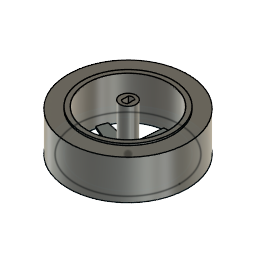
chassis_v1 (Autodesk Fusion 360 archive; units mm, degrees)
design "BO_Wheel"
part number: 2025-11-15-17-17-48-171
Autodesk Fusion 360 part; units mm, degrees
note: some values were not read from the file. Set by a fixed rule: which face or edge a step refers to.
sketch "Sketch1" plane through (0, 0, 0) normal (0, 0, 1) x (1, 0, 0)
  circle A0 centre (0, 0) radius 23.675
  circle A1 centre (0, 0) radius 23.175
  dimension "d1" = 47.35
  dimension "d2" = 46.35
  constraint coincident A0.centre A1.centre
  measures "d1" diameter of A0
  measures "d2" diameter of A1
extrude "Extrude1" add sketch "Sketch1" along normal blind 24.4 makes body 1
sketch "Sketch2" plane through (0, 0, 24.4) normal (0, 0, 1) x (-1, 0, 0)
  circle A0 centre (0, 0) radius 23.175
  circle A1 centre (0, 0) radius 23.675
  circle A2 centre (0, 0) radius 25.7
  dimension "d5" = 51.4
  constraint concentric A0 A2
  measures "d5" diameter of A2
extrude "Extrude2" add sketch "Sketch2" against normal blind 1 contours A1 | A2 bodies 1
mirror "Mirror1" about plane through (0, 0, 12.2) normal (0, 0, -1) of bodies 1 merged
sketch "Sketch3" plane through (0, 0, 1) normal (0, 0, 1) x (-1, 0, 0)
  circle A0 centre (0, 0) radius 25.7
  circle A1 centre (0, 0) radius 23.675
  circle A2 centre (0, 0) radius 33.8
  dimension "d10" = 67.6
  constraint coincident A0.centre A1.centre
  measures "d10" diameter of A2
extrude "Extrude3" add sketch "Sketch3" along normal blind 22.4 separate body contours A2 makes body 2
sketch "Sketch4" plane through (0, 0, 0) normal (0, 0, -1) x (1, 0, 0)
  circle A0 centre (0, 0) radius 25.7
  circle A1 centre (0, 0) radius 23.175
  circle A2 centre (0, 0) radius 4.56
  dimension "d13" = 9.12
  constraint concentric A0 A2
  measures "d13" diameter of A2
extrude "Extrude4" add sketch "Sketch4" against normal blind 27.7 separate body contours A2 makes body 3
extrude "Extrude5" cut 1 faces at (-0.7219, -0.8073, 0) along direction (0, 0, 1) blind 4.3 on bodies 3 bodies 3
sketch "Sketch5" plane through (0, 0, 4.3) normal (0, 0, -1) x (1, 0, 0)
  circle A0 centre (0, 0) radius 4.56
  circle A1 centre (0, 0) radius 7.16
  circle A2 centre (0, 0) radius 4.56
  dimension "d18" = 14.32
  constraint concentric A0 A1
  constraint concentric A1 A2
  measures "d18" diameter of A1
extrude "Extrude6" add sketch "Sketch5" along normal blind 1 separate body makes body 4
extrude "Extrude7" add 1 faces at (-0.7219, -0.8073, 4.3) along direction (0, 0, -1) blind 2 on bodies 3 bodies 3 4
sketch "Sketch6" plane through (0, 0, 0) normal (0, 0, -1) x (1, 0, 0)
  circle A0 centre (0, 0) radius 25.7
  circle A1 centre (0, 0) radius 23.175
  circle A2 centre (0, 0) radius 9.19
  line L0 (0, -23.175) -> (22.0407, -7.1615)
  line L1 (22.0407, -7.1615) -> (13.6219, 18.749)
  line L2 (13.6219, 18.749) -> (-13.6219, 18.749)
  line L3 (-13.6219, 18.749) -> (-22.0407, -7.1615)
  line L4 (-22.0407, -7.1615) -> (0, -23.175)
  line L5 (2.8, -23.6825) -> (-2.8, -23.6825)
  line L6 (2.8, -23.6825) -> (-2.8, -8.6825) construction
  line L7 (-2.8, -23.6825) -> (2.8, -8.6825) construction
  line L8 (4.07, -9.19) -> (2.8, -23.0052)
  line L9 (-2.8, -23.0052) -> (-4.07, -9.19)
  line L10 (-4.07, -9.19) -> (-4.1616, -8.1937)
  line L11 (4.07, -9.19) -> (4.1616, -8.1937)
  circle A3 centre (0, 0) radius 7.161
  point P0 (0, -16.1825)
  point P1 (0, -16.1825)
  dimension "d23" = 18.38
  dimension "d24" = 5.6
  dimension "d25" = 15
  constraint concentric A0 A2
  constraint coincident A1 L0.start
  constraint coincident A0.centre A1.centre
  constraint horizontal L5
  constraint coincident L6 P1
  constraint coincident L7 P1
  constraint coincident P1 P0
  constraint coincident A1 L8.end
  constraint coincident A1 L9.start
  constraint coincident A2 L10.end
  constraint parallel L9 L10
  constraint coincident A2 L11.end
  constraint parallel L8 L11
  measures "d23" diameter of A2
  measures "d24" distance of L6.end L7.end
  measures "d25" distance of L5.end L6.end
extrude "Extrude8" add sketch "Sketch6" against normal blind 1 contours A1 L0 L8 | A2 L0 L4 L8 L9 L10 L11 | A1 L4 L9 | A2 picked at (2.551, -22.3707) picked at (-2.551, -22.3707) bodies 1
pattern_circular "C-Pattern1" count 5 over 360 about axis through (0, 0, 1.75) along (0, 0, 1) of bodies 1 makes body 5 at (-16.9051, 5.3053, 0) makes body 6 at (-10.5582, -14.2286, 0) makes body 7 at (10.2696, -14.4383, 0) makes body 8 at (16.7949, 5.6446, 0)
sketch "Sketch7" plane through (0, 0, 1) normal (0, 0, -1) x (1, 0, 0)
  circle A0 centre (0, 0) radius 25.7
  circle A1 centre (0, 0) radius 33.8
  circle A2 centre (0, 0) radius 29.25
  dimension "d32" = 58.5
  constraint concentric A0 A2
  measures "d32" diameter of A2
sketch "Sketch8" plane through (0, 0, 27.7) normal (0, 0, 1) x (-1, 0, 0)
  circle A0 centre (0, 0) radius 4.56
  line L0 (1.78, 0) -> (1.78, -2.03)
  line L1 (1.78, 0) -> (1.78, 2.03)
  line L2 (-1.78, 0) -> (-1.78, -2.03)
  line L3 (-1.78, 0) -> (-1.78, 2.03)
  circle A1 centre (0, 0) radius 2.6999
  circle A2 centre (0, 0) radius 0.98
  dimension "d33" = 1.78
  dimension "d34" = 2.03
  dimension "d35" = 2.03
  dimension "d36" = 1.78
  dimension "d37" = 2.03
  dimension "d39" = 2.03
  dimension "d40" = 1.96
  constraint coincident A0.centre A1.centre
  constraint coincident L0.end A1
  constraint concentric A1 A2
  measures "d33" distance of A0.centre L0.start
  measures "d34" distance of L0.start L0.end
  measures "d35" distance of L0.start L1.end
  measures "d36" distance of A0.centre L2.start
  measures "d37" distance of L2.start L2.end
  measures "d39" distance of L2.start L3.end
  measures "d40" diameter of A2
extrude "Extrude9" cut sketch "Sketch8" against normal blind 8 contours L0 L1 L2 L3 A1 | A2 bodies 3

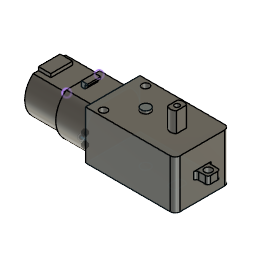
design "BO_Motor"
part number: 2025-11-14-23-14-41-940
Autodesk Fusion 360 part; units mm, degrees
sketch "Sketch1" plane through (0, 0, 0) normal (0, 0, 1) x (1, 0, 0)
  line L0 (-18.1, 11) -> (18.1, 11)
  line L1 (18.1, 11) -> (18.1, -11)
  line L2 (18.1, -11) -> (-18.1, -11)
  line L3 (-18.1, -11) -> (-18.1, 11)
  line L4 (-18.1, 11) -> (18.1, -11) construction
  line L5 (18.1, 11) -> (-18.1, -11) construction
  dimension "d1" = 36.2
  dimension "d2" = 22
  constraint horizontal L0
  constraint perpendicular L0 L1
  constraint parallel L0 L2
  constraint parallel L1 L3
  constraint coincident L4 origin
  constraint coincident L5 origin
  measures "d1" distance of L1.end L2.end
  measures "d2" distance of L0.end L1.end
extrude "Extrude1" add sketch "Sketch1" along normal blind 19.6 makes body 1
sketch "Sketch2" plane through (0, 0, 19.6) normal (0, 0, 1) x (-1, 0, 0)
  line L0 (18.1, 11) -> (-18.1, 11)
  line L1 (-18.1, 11) -> (-18.1, -11)
  line L2 (-18.1, -11) -> (18.1, -11)
  line L3 (18.1, -11) -> (18.1, 11)
  circle A0 centre (-7.88, 0) radius 2.7
  line L4 (-6.1, 0) -> (-6.1, -2.0302)
  line L5 (-6.1, 0) -> (-6.1, 2.0302)
  line L6 (-9.66, 0) -> (-9.66, -2.0302)
  line L7 (-9.66, 2.0302) -> (-9.66, 0)
  circle A1 centre (-7.88, 0) radius 0.98
  point P0 (-7.88, 0)
  point P1 (-6.1, 0)
  point P2 (-9.66, 0)
  dimension "d6" = 3.56
  dimension "d8" = 5.4
  constraint coincident P0 A0.centre
  constraint coincident P1 L4.start
  constraint coincident A0 L4.end
  constraint vertical L4
  constraint coincident A0 L5.end
  constraint parallel L4 L5
  constraint coincident P2 L6.start
  constraint coincident A0 L6.end
  constraint vertical L6
  constraint coincident A0 L7.start
  constraint parallel L6 L7
  measures "d6" distance of P1 P2
  measures "d8" diameter of A0
extrude "Extrude2" add sketch "Sketch2" along normal blind 8 contours A0 L4 L5 L6 L7 bodies 1
sketch "Sketch3" plane through (0, 0, 19.6) normal (0, 0, 1) x (-1, 0, 0)
  line L0 (18.1, 11) -> (-18.1, 11)
  line L1 (-18.1, 11) -> (-18.1, -11)
  line L2 (-18.1, -11) -> (18.1, -11)
  line L3 (18.1, -11) -> (18.1, 11)
  arc A0 (-9.66, -2.0302) -> (-6.1, -2.0302) centre (-7.88, 0) ccw
  line L4 (-9.66, -2.0302) -> (-9.66, 2.0302)
  arc A1 (-6.1, 2.0302) -> (-9.66, 2.0302) centre (-7.88, 0) ccw
  line L5 (-6.1, 2.0302) -> (-6.1, -2.0302)
  circle A2 centre (4.79, 0) radius 1.91
extrude "Extrude3" add sketch "Sketch3" along normal blind 1.1 contours A2 bodies 1
mirror "Mirror1" about plane through (0, 0, 9.8) normal (0, 0, 1) of bodies 1 merged
sketch "Sketch4" plane through (0, 0, 0) normal (0, 0, -1) x (1, 0, 0)
  line L0 (18.1, 11) -> (-18.1, 11)
  line L1 (-18.1, 11) -> (-18.1, -11)
  line L2 (-18.1, -11) -> (18.1, -11)
  line L3 (18.1, -11) -> (18.1, 11)
  arc A0 (6.1, -2.0302) -> (9.66, -2.0302) centre (7.88, 0) ccw
  line L4 (6.1, -2.0302) -> (6.1, 2.0302)
  arc A1 (9.66, 2.0302) -> (6.1, 2.0302) centre (7.88, 0) ccw
  line L5 (9.66, 2.0302) -> (9.66, -2.0302)
  circle A2 centre (-4.79, 0) radius 1.91
extrude "Extrude4" cut 1 faces at (-4.2895, 0.234, -1.1) along direction (0, 0, 1) blind 1.1 on bodies 1 bodies 1
sketch "Sketch5" plane through (18.1, 0, 0) normal (1, 0, 0) x (0, 1, 0)
  line L0 (-11, 0) -> (11, 0)
  line L1 (11, 0) -> (11, 19.6)
  line L2 (11, 19.6) -> (-11, 19.6)
  line L3 (-11, 19.6) -> (-11, 0)
  line L4 (0, 0) -> (0, 9.8)
  line L5 (-2.5, 11.3) -> (2.5, 11.3)
  line L6 (2.5, 11.3) -> (2.5, 8.3)
  line L7 (2.5, 8.3) -> (-2.5, 8.3)
  line L8 (-2.5, 8.3) -> (-2.5, 11.3)
  line L9 (-2.5, 11.3) -> (2.5, 8.3) construction
  line L10 (2.5, 11.3) -> (-2.5, 8.3) construction
  point P0 (0, 9.8)
  dimension "d20" = 9.8
  dimension "d21" = 5
  dimension "d22" = 3
  constraint coincident L4.start origin
  constraint perpendicular L2 L4
  constraint horizontal L5
  constraint perpendicular L5 L6
  constraint parallel L5 L7
  constraint parallel L6 L8
  constraint coincident L9 P0
  constraint coincident L10 P0
  constraint coincident P0 L4.end
  measures "d20" distance of L4.start P0
  measures "d21" distance of L6.end L7.end
  measures "d22" distance of L5.end L6.end
extrude "Extrude5" add sketch "Sketch5" along normal blind 4.76 contours L5 L6 L7 L8 bodies 1
sketch "Sketch6" plane through (0, 0, 11.3) normal (0, 0, 1) x (-1, 0, 0)
  line L0 (-18.1, -2.5) -> (-18.1, 2.5)
  line L1 (-18.1, 2.5) -> (-22.86, 2.5)
  line L2 (-22.86, 2.5) -> (-22.86, -2.5)
  line L3 (-22.86, -2.5) -> (-18.1, -2.5)
  line L4 (-22.86, 0) -> (-20.48, 0)
  circle A0 centre (-20.48, 0) radius 1.5
  dimension "d25" = 2.38
  dimension "d26" = 3
  constraint midpoint L2 L4.start
  constraint perpendicular L0 L4
  constraint coincident L4.end A0.centre
  measures "d25" distance of L4.start L4.end
  measures "d26" diameter of A0
extrude "Extrude6" cut sketch "Sketch6" against normal blind 3 contours A0 bodies 1
sketch "Sketch7" plane through (0, 0, 11.3) normal (0, 0, 1) x (-1, 0, 0)
  circle A0 centre (-20.48, 0) radius 1.5
  line L0 (-18.1, -2.5) -> (-18.1, 2.5)
  line L1 (-18.1, 2.5) -> (-22.86, 2.5)
  line L2 (-22.86, 2.5) -> (-22.86, -2.5)
  line L3 (-22.86, -2.5) -> (-18.1, -2.5)
  line L4 (-22.86, -2.5) -> (-21.86, -2.5)
  line L5 (-21.86, -2.5) -> (-21.86, -1.5)
  line L6 (-21.86, -1.5) -> (-22.86, -1.5)
  line L7 (-22.86, -1.5) -> (-22.86, -2.5)
  line L8 (-22.86, 2.5) -> (-21.86, 2.5)
  line L9 (-21.86, 2.5) -> (-21.86, 1.5)
  line L10 (-21.86, 1.5) -> (-22.86, 1.5)
  line L11 (-22.86, 1.5) -> (-22.86, 2.5)
  circle A1 centre (-21.86, 1.5) radius 1
  circle A2 centre (-21.86, -1.5) radius 1
  line L12 (-18.1, -2.5) -> (-19.1, -2.5)
  line L13 (-19.1, -2.5) -> (-19.1, -3.5)
  line L14 (-19.1, -3.5) -> (-18.1, -3.5)
  line L15 (-18.1, -3.5) -> (-18.1, -2.5)
  line L16 (-18.1, 2.5) -> (-19.1, 2.5)
  line L17 (-19.1, 2.5) -> (-19.1, 3.5)
  line L18 (-19.1, 3.5) -> (-18.1, 3.5)
  line L19 (-18.1, 3.5) -> (-18.1, 2.5)
  circle A3 centre (-19.1, 3.5) radius 1
  circle A4 centre (-19.1, -3.5) radius 1
  dimension "d29" = 1
  dimension "d30" = 1
  dimension "d31" = 1
  dimension "d32" = 1
  dimension "d33" = 1
  dimension "d34" = 1
  dimension "d35" = 1
  dimension "d36" = 1
  constraint horizontal L4
  constraint vertical L5
  constraint horizontal L6
  constraint vertical L7
  constraint coincident L2.end L3.start
  constraint horizontal L8
  constraint vertical L9
  constraint horizontal L10
  constraint vertical L11
  constraint coincident L1.end L2.start
  constraint coincident L9.end L10.start
  constraint coincident L10.end A1
  constraint coincident L5.end L6.start
  constraint coincident L4.end A2
  constraint horizontal L12
  constraint vertical L13
  constraint horizontal L14
  constraint vertical L15
  constraint coincident L0.start L3.end
  constraint horizontal L16
  constraint vertical L17
  constraint horizontal L18
  constraint vertical L19
  constraint coincident L0.end L1.start
  constraint coincident L17.end L18.start
  constraint coincident L18.end A3
  constraint coincident L13.end L14.start
  constraint coincident L12.end A4
  measures "d29" distance of L2.end L4.end
  measures "d30" distance of L2.end L6.end
  measures "d31" distance of L1.end L8.end
  measures "d32" distance of L1.end L10.end
  measures "d33" distance of L0.start L12.end
  measures "d34" distance of L0.start L14.end
  measures "d35" distance of L0.end L16.end
  measures "d36" distance of L0.end L18.end
extrude "Extrude7" cut sketch "Sketch7" against normal blind 3 contours L1 L2 L8 L11 A1 | L2 L3 L4 L7 A2 | L1 L16 L19 A3 | L3 L12 L15 A4 bodies 1
sketch "Sketch8" plane through (0, 0, 11.3) normal (0, 0, 1) x (-1, 0, 0)
  circle A0 centre (-20.48, 0) radius 1.5
  arc A1 (-22.86, -1.5) -> (-21.86, -2.5) centre (-21.86, -1.5) ccw
  line L0 (-21.86, -2.5) -> (-18.1, -2.5)
  line L1 (-18.1, -2.5) -> (-18.1, 2.5)
  line L2 (-18.1, 2.5) -> (-21.86, 2.5)
  arc A2 (-21.86, 2.5) -> (-22.86, 1.5) centre (-21.86, 1.5) ccw
  line L3 (-22.86, 1.5) -> (-22.86, -1.5)
  line L4 (-18.1, -2.5) -> (-19.1, -2.5)
  line L5 (-19.1, -2.5) -> (-19.1, -3.5)
  line L6 (-19.1, -3.5) -> (-18.1, -3.5)
  line L7 (-18.1, -3.5) -> (-18.1, -2.5)
  line L8 (-18.1, 2.5) -> (-19.1, 2.5)
  line L9 (-19.1, 2.5) -> (-19.1, 3.5)
  line L10 (-19.1, 3.5) -> (-18.1, 3.5)
  line L11 (-18.1, 3.5) -> (-18.1, 2.5)
  circle A3 centre (-19.1, -3.5) radius 1
  circle A4 centre (-19.1, 3.5) radius 1
  dimension "d39" = 1
  dimension "d40" = 1
  dimension "d41" = 1
  dimension "d42" = 1
  constraint horizontal L4
  constraint vertical L5
  constraint horizontal L6
  constraint vertical L7
  constraint coincident L0.end L1.start
  constraint horizontal L8
  constraint vertical L9
  constraint horizontal L10
  constraint vertical L11
  constraint coincident L1.end L2.start
  constraint coincident L5.end L6.start
  constraint coincident L4.end A3
  constraint coincident L9.end L10.start
  constraint coincident L8.end A4
  measures "d39" distance of L0.end L4.end
  measures "d40" distance of L0.end L6.end
  measures "d41" distance of L1.end L8.end
  measures "d42" distance of L1.end L10.end
extrude "Extrude8" add sketch "Sketch8" against normal blind 3 contours L0 L4 L7 A3 | L2 L8 L11 A4 bodies 1
sketch "Sketch9" plane through (0, 0, 19.6) normal (0, 0, 1) x (-1, 0, 0)
  circle A0 centre (4.79, 0) radius 1.91
  line L0 (18.1, 11) -> (-18.1, 11)
  line L1 (-18.1, 11) -> (-18.1, -11)
  line L2 (-18.1, -11) -> (18.1, -11)
  line L3 (18.1, -11) -> (18.1, 11)
  arc A1 (-9.66, -2.0302) -> (-6.1, -2.0302) centre (-7.88, 0) ccw
  line L4 (-9.66, -2.0302) -> (-9.66, 2.0302)
  arc A2 (-6.1, 2.0302) -> (-9.66, 2.0302) centre (-7.88, 0) ccw
  line L5 (-6.1, 2.0302) -> (-6.1, -2.0302)
  line L6 (-18.1, -11) -> (-16.1, -11)
  line L7 (-16.1, -11) -> (-16.1, -9)
  line L8 (-16.1, -9) -> (-18.1, -9)
  line L9 (-18.1, -9) -> (-18.1, -11)
  line L10 (-18.1, 11) -> (-16.1, 11)
  line L11 (-16.1, 11) -> (-16.1, 9)
  line L12 (-16.1, 9) -> (-18.1, 9)
  line L13 (-18.1, 9) -> (-18.1, 11)
  circle A3 centre (-16.1, -9) radius 2
  circle A4 centre (-16.1, 9) radius 2
  dimension "d45" = 2
  dimension "d46" = 2
  dimension "d47" = 2
  dimension "d48" = 2
  constraint horizontal L6
  constraint vertical L7
  constraint horizontal L8
  constraint vertical L9
  constraint coincident L1.end L2.start
  constraint horizontal L10
  constraint vertical L11
  constraint horizontal L12
  constraint vertical L13
  constraint coincident L0.end L1.start
  constraint coincident L7.end L8.start
  constraint coincident L6.end A3
  constraint coincident L11.end L12.start
  constraint coincident L10.end A4
  measures "d45" distance of L1.end L6.end
  measures "d46" distance of L1.end L8.end
  measures "d47" distance of L0.end L10.end
  measures "d48" distance of L0.end L12.end
extrude "Extrude9" cut sketch "Sketch9" against normal blind 19.6 contours L0 L1 L10 L13 A4 | L1 L2 L6 L9 A3 bodies 1
sketch "Sketch10" plane through (-18.1, 0, 0) normal (-1, 0, 0) x (0, -1, 0)
  line L0 (-11, 0) -> (11, 0)
  line L1 (11, 0) -> (11, 19.6)
  line L2 (11, 19.6) -> (-11, 19.6)
  line L3 (-11, 19.6) -> (-11, 0)
  line L4 (0, 0) -> (-6.875, 0)
  line L5 (0, 0) -> (6.875, 0)
  line L6 (0, 0) -> (0, 17.4)
  line L7 (0, 0) -> (0, 8.7)
  line L8 (0, 17.4) -> (-6.875, 17.4)
  line L9 (0, 17.4) -> (6.875, 17.4)
  circle A0 centre (0, 8.7) radius 11
  circle A1 centre (0, 8.7) radius 10
  line L10 (0, 17.4) -> (0, 16.4)
  line L11 (0, 0) -> (0, 1)
  line L12 (0, 0) -> (0, 1)
  line L13 (0, 1) -> (7.8556, 1)
  line L14 (0, 1) -> (-7.8556, 1)
  line L15 (0, 16.4) -> (7.8556, 16.4)
  line L16 (0, 16.4) -> (-7.8556, 16.4)
  dimension "d51" = 6.875
  dimension "d52" = 6.875
  dimension "d53" = 17.4
  dimension "d54" = 8.7
  dimension "d55" = 6.875
  dimension "d56" = 6.875
  dimension "d57" = 20
  dimension "d58" = 1
  dimension "d59" = 1
  constraint coincident L4.start L5.start
  constraint parallel L0 L4
  constraint perpendicular L3 L5
  constraint vertical L6
  constraint perpendicular L0 L7
  constraint perpendicular L6 L8
  constraint perpendicular L6 L9
  constraint coincident L7.end A0.centre
  constraint tangent L3 A0
  constraint perpendicular L8 L10
  constraint coincident L7 L11.end
  constraint perpendicular L4 L12
  constraint coincident A0 L13.end
  constraint perpendicular L7 L13
  constraint coincident A0 L14.end
  constraint perpendicular L11 L14
  constraint coincident A0 L15.end
  constraint perpendicular L10 L15
  constraint coincident A0 L16.end
  constraint perpendicular L6 L16
  measures "d51" distance of L4.start L4.end
  measures "d52" distance of L4.start L5.end
  measures "d53" distance of L4.start L6.end
  measures "d54" distance of L4.start L7.end
  measures "d55" distance of L6.end L8.end
  measures "d56" distance of L6.end L9.end
  measures "d57" diameter of A1
  measures "d58" distance of L6.end L10.end
  measures "d59" distance of L4.start L11.end
extrude "Extrude10" add sketch "Sketch10" along normal blind 12.04 contours A0 A1 L14 L16 | L0 L4 A0 A1 L14 | L8 A0 A1 L16 | L0 L4 L6 L7 A1 L11 L12 L14 | L0 L5 A0 A1 L13 | L6 L8 A1 L10 L16 | L0 L5 L6 L7 A1 L11 L12 L13 | A0 A1 L13 L15 | L6 L9 A1 L10 L15 | L9 A0 A1 L15 bodies 1
extrude "Extrude11" add 1 faces at (-18.1, 2.9458, 13.0089) along direction (-1, 0, 0) blind 12.04 on bodies 1 bodies 1
sketch "Sketch11" plane through (-30.14, 0, 0) normal (-1, 0, 0) x (0, -1, 0)
  line L0 (-6.7313, 0) -> (6.7313, 0)
  arc A0 (6.7313, 0) -> (6.7313, 17.4) centre (0, 8.7) ccw
  line L1 (6.7313, 17.4) -> (-6.7313, 17.4)
  arc A1 (-6.7313, 17.4) -> (-6.7313, 0) centre (0, 8.7) ccw
  line L2 (0, 8.7) -> (-9.95, 8.7)
  line L3 (0, 8.7) -> (9.95, 8.7)
  line L4 (0, 8.7) -> (0, 16.2)
  line L5 (0, 8.7) -> (0, 1.2)
  line L6 (0, 1.2) -> (-11, 1.2)
  line L7 (-11, 1.2) -> (11, 1.2)
  line L8 (11, 1.2) -> (11, 16.2)
  line L9 (11, 16.2) -> (0, 16.2)
  line L10 (0, 16.2) -> (-11, 16.2)
  line L11 (-11, 16.2) -> (-11, 1.2)
  circle A2 centre (0, 8.7) radius 9.95
  point P0 (0, 8.7)
  dimension "d64" = 9.95
  dimension "d65" = 9.95
  dimension "d66" = 7.5
  dimension "d67" = 7.5
  constraint coincident P0 A0.centre
  constraint horizontal L2
  constraint parallel L2 L3
  constraint perpendicular L3 L4
  constraint perpendicular L3 L5
  constraint perpendicular L5 L6
  constraint parallel L6 L7
  constraint perpendicular L3 L8
  constraint perpendicular L4 L9
  constraint perpendicular L4 L10
  constraint perpendicular L6 L11
  constraint coincident L2.end A2
  measures "d64" distance of P0 L2.end
  measures "d65" distance of P0 L3.end
  measures "d66" distance of P0 L4.end
  measures "d67" distance of P0 L5.end
extrude "Extrude12" add sketch "Sketch11" along normal blind 8.65 contours L2 L5 L6 L7 A2 | L3 L5 L7 A2 | L2 L4 L10 A2 | L3 L4 L9 A2 bodies 1
sketch "Sketch12" plane through (0, 0, 16.2) normal (0, 0, 1) x (-1, 0, 0)
  line L0 (30.14, 6.5385) -> (30.14, -6.5385)
sketch "Sketch13" plane through (-38.79, 0, 0) normal (-1, 0, 0) x (0, -1, 0)
  arc A0 (6.5385, 1.2) -> (6.5385, 16.2) centre (0, 8.7) ccw
  line L0 (6.5385, 16.2) -> (-6.5385, 16.2)
  arc A1 (-6.5385, 16.2) -> (-6.5385, 1.2) centre (0, 8.7) ccw
  line L1 (-6.5385, 1.2) -> (6.5385, 1.2)
  point P0 (0, 17.65)
sketch "Sketch14" plane through (0, 0, 16.2) normal (0, 0, 1) x (-1, 0, 0)
sketch "Sketch15" plane through (-38.79, 0, 0) normal (-1, 0, 0) x (0, -1, 0)
extrude "Extrude13" add sketch "Sketch13" along normal blind 4.96 bodies 1
sketch "Sketch16" plane through (0, 0, 16.2) normal (0, 0, 1) x (-1, 0, 0)
  line L0 (30.14, 6.5385) -> (30.14, -6.5385)
  line L1 (30.14, -6.5385) -> (43.75, -6.5385)
  line L2 (43.75, -6.5385) -> (43.75, 6.5385)
  line L3 (43.75, 6.5385) -> (30.14, 6.5385)
  line L4 (43.75, 0) -> (41.25, 0)
  line L5 (43.75, -4.4) -> (38.75, -4.4)
  line L6 (38.75, -4.4) -> (38.75, 4.4)
  line L7 (38.75, 4.4) -> (43.75, 4.4)
  line L8 (43.75, 4.4) -> (43.75, -4.4)
  line L9 (43.75, -4.4) -> (38.75, 4.4) construction
  line L10 (38.75, -4.4) -> (43.75, 4.4) construction
  point P0 (41.25, 0)
  dimension "d74" = 5
  dimension "d75" = 8.8
  constraint midpoint L2 L4.start
  constraint horizontal L5
  constraint perpendicular L5 L6
  constraint parallel L5 L7
  constraint parallel L6 L8
  constraint coincident L9 P0
  constraint coincident L10 P0
  constraint coincident P0 L4.end
  measures "d74" distance of L6.end L7.end
  measures "d75" distance of L5.end L6.end
extrude "Extrude14" add sketch "Sketch16" along normal blind 1.4 contours L2 L5 L6 L7 L8 bodies 1
sketch "Sketch17" plane through (0, 0, 20.7) normal (0, 0, 1) x (-1, 0, 0)
  circle A0 centre (4.79, 0) radius 1.91
sketch "Sketch18" plane through (-18.1, 0, 0) normal (-1, 0, 0) x (0, -1, 0)
  arc A0 (11, 8.7) -> (6.7313, 17.4) centre (0, 8.7) ccw
  line L0 (11, 8.7) -> (11, 19.6)
  line L1 (11, 19.6) -> (-11, 19.6)
  line L2 (-11, 19.6) -> (-11, 8.7)
  arc A1 (-6.7313, 17.4) -> (-11, 8.7) centre (0, 8.7) ccw
  line L3 (-6.7313, 17.4) -> (6.7313, 17.4)
sketch "Sketch19" plane through (0, 0, 17.4) normal (0, 0, 1) x (-1, 0, 0)
  line L0 (18.1, 6.7313) -> (18.1, -6.7313)
  line L1 (18.1, -6.7313) -> (30.14, -6.7313)
  line L2 (30.14, -6.7313) -> (30.14, 6.7313)
  line L3 (30.14, 6.7313) -> (18.1, 6.7313)
  line L4 (18.1, 0) -> (28.09, 0)
  line L5 (28.09, 0) -> (28.09, -2.65)
  line L6 (28.09, 0) -> (28.09, 2.65)
  line L7 (28.09, 0) -> (25.64, 0)
  line L8 (28.09, -2.65) -> (25.64, -2.65)
  line L9 (25.64, -2.65) -> (25.64, 2.65)
  line L10 (25.64, 2.65) -> (28.09, 2.65)
  line L11 (28.09, 2.65) -> (28.09, -2.65)
  dimension "d79" = 2.65
  dimension "d80" = 2.65
  dimension "d81" = 2.45
  dimension "d82" = 2.45
  dimension "d83" = 5.3
  constraint midpoint L0 L4.start
  constraint perpendicular L0 L4
  constraint perpendicular L4 L5
  constraint perpendicular L4 L6
  constraint perpendicular L5 L7
  constraint horizontal L8
  constraint vertical L9
  constraint horizontal L10
  constraint vertical L11
  measures "d79" distance of L4.end L5.end
  measures "d80" distance of L4.end L6.end
  measures "d81" distance of L4.end L7.end
  measures "d82" distance of L5.end L8.end
  measures "d83" distance of L5.end L6.end
extrude "Extrude15" add sketch "Sketch19" along normal blind 2.175 separate body contours L4 L6 L7 L9 L10 L11 | L4 L5 L7 L8 L9 L11 makes body 2
mirror "Mirror2" about plane through (0, 0, 9.8) normal (0, 0, 1) of bodies 2 makes body 3
extrude "Extrude16" add 1 faces at (-26.4567, 0.8833, 0.025) along direction (0, 0, -1) blind 2.175 on bodies 3 bodies 3
sketch "Sketch20" plane through (0, -2.65, 0) normal (0, -1, 0) x (1, 0, 0)
  line L0 (-28.09, 17.4) -> (-25.64, 17.4)
  line L1 (-25.64, 17.4) -> (-25.64, 19.575)
  line L2 (-25.64, 19.575) -> (-28.09, 19.575)
  line L3 (-28.09, 19.575) -> (-28.09, 17.4)
  line L4 (-28.09, 17.4) -> (-26.64, 17.4)
  line L5 (-26.64, 17.4) -> (-26.64, 18.85)
  line L6 (-26.64, 18.85) -> (-25.64, 18.85)
  dimension "d90" = 1.45
  dimension "d91" = 1.45
  constraint coincident L0.start L3.end
  constraint perpendicular L1 L4
  constraint perpendicular L0 L5
  constraint coincident L1 L6.end
  constraint perpendicular L1 L6
  measures "d90" distance of L0.start L4.end
  measures "d91" distance of L4.end L5.end
extrude "Extrude17" cut sketch "Sketch20" against normal blind 6 contours L0 L1 L5 L6 bodies 2
sketch "Sketch21" plane through (0, -2.65, 0) normal (0, -1, 0) x (1, 0, 0)
  line L0 (-25.64, 2.2) -> (-28.09, 2.2)
  line L1 (-28.09, 2.2) -> (-28.09, -2.15)
  line L2 (-28.09, -2.15) -> (-25.64, -2.15)
  line L3 (-25.64, -2.15) -> (-25.64, 2.2)
  line L4 (-28.09, -0.2126) -> (-26.64, -0.2126)
  line L5 (-26.64, -0.2126) -> (-26.64, 2.2)
  line L6 (-26.64, -0.2126) -> (-26.64, -2.15)
  dimension "d94" = 1.45
  constraint coincident L1 L4.start
  constraint perpendicular L1 L4
  constraint coincident L0 L5.end
  constraint perpendicular L0 L5
  constraint coincident L2 L6.end
  constraint perpendicular L2 L6
  measures "d94" distance of L4.start L4.end
sketch "Sketch22" plane through (0, -2.65, 0) normal (0, -1, 0) x (1, 0, 0)
  line L0 (-26.64, 17.4) -> (-26.64, 18.85)
  line L1 (-26.64, 18.85) -> (-25.64, 18.85)
  line L2 (-25.64, 18.85) -> (-25.64, 19.575)
  line L3 (-25.64, 19.575) -> (-28.09, 19.575)
  line L4 (-28.09, 19.575) -> (-28.09, 17.4)
  line L5 (-28.09, 17.4) -> (-26.64, 17.4)
sketch "Sketch23" plane through (0, -2.65, 0) normal (0, -1, 0) x (1, 0, 0)
  line L0 (-26.64, -2.15) -> (-26.64, -1.425)
  line L1 (-26.64, -1.425) -> (-25.6393, -1.425)
  line L2 (-25.6393, -1.425) -> (-25.6393, 0)
  line L3 (-25.6393, 0) -> (-26.64, 0)
  line L4 (-26.64, 0) -> (-25.6393, 0)
  line L5 (-25.6393, 0) -> (-25.6393, -1.425)
  line L6 (-25.6393, -1.425) -> (-26.64, -1.425)
  line L7 (-26.64, -1.425) -> (-26.64, 0)
  dimension "d95" = 0.725
  constraint vertical L0
  constraint perpendicular L0 L1
  constraint perpendicular L1 L2
  constraint perpendicular L2 L3
  constraint perpendicular L3 L7
  measures "d95" distance of L0.start L0.end
extrude "Extrude18" cut sketch "Sketch23" against normal blind 6 bodies 3
sketch "Sketch24" plane through (-43.75, 0, 0) normal (-1, 0, 0) x (0, -1, 0)
  line L0 (-6.5385, 1.2) -> (6.5385, 1.2)
  arc A0 (6.5385, 1.2) -> (6.5385, 16.2) centre (0, 8.7) ccw
  line L1 (6.5385, 16.2) -> (4.4, 16.2)
  line L2 (4.4, 16.2) -> (4.4, 17.6)
  line L3 (4.4, 17.6) -> (-4.4, 17.6)
  line L4 (-4.4, 17.6) -> (-4.4, 16.2)
  line L5 (-4.4, 16.2) -> (-6.5385, 16.2)
  arc A1 (-6.5385, 16.2) -> (-6.5385, 1.2) centre (0, 8.7) ccw
  line L6 (0, 1.2) -> (0, 17.6)
  line L7 (-4.4, 16.2) -> (4.4, 16.2)
  line L8 (0, 16.2) -> (0, 8.7)
  circle A2 centre (0, 8.7) radius 4.925
  line L9 (0, 13.625) -> (0, 4.825)
  line L10 (0, 4.825) -> (-3.0397, 4.825)
  line L11 (0, 4.825) -> (3.0397, 4.825)
  dimension "d98" = 9.85
  dimension "d99" = 8.8
  constraint midpoint L0 L6.start
  constraint midpoint L3 L6.end
  constraint coincident L4.end L5.start
  constraint coincident L1.end L2.start
  constraint midpoint L7 L8.start
  constraint coincident A0.centre A1.centre
  constraint coincident A2 L9.start
  constraint coincident L8 L9.start
  constraint parallel L6 L9
  constraint coincident A2 L10.end
  constraint perpendicular L6 L10
  constraint coincident A2 L11.end
  constraint perpendicular L6 L11
  measures "d98" diameter of A2
  measures "d99" distance of L9.start L9.end
extrude "Extrude19" add sketch "Sketch24" along normal blind 2.35 contours L6 L8 A2 L9 L10 | L6 L8 A2 L9 L11 bodies 1
sketch "Sketch25" plane through (-46.1, 0, 0) normal (-1, 0, 0) x (0, -1, 0)
  line L0 (-3.0397, 4.825) -> (3.0397, 4.825)
  arc A0 (3.0397, 4.825) -> (-3.0397, 4.825) centre (0, 8.7) ccw
  line L1 (4.3381, 6.3684) -> (-4.3381, 11.0316)
  circle A1 centre (0, 8.7) radius 1
  dimension "d102" = 9.85
  dimension "d103" = 2
  constraint coincident A0 L1.start
  constraint coincident A0 L1.end
  constraint concentric A0 A1
  measures "d102" distance of L1.start L1.end
  measures "d103" diameter of A1
extrude "Extrude20" add sketch "Sketch25" along normal blind 0.65 contours L1 A1 | L1 A1 bodies 1
sketch "Sketch26" plane through (0, 0, 0) normal (0, 1, 0) x (1, 0, 0)
sketch "Sketch27" plane through (0, 0, 19.6) normal (0, 0, 1) x (-1, 0, 0)
  arc A0 (-16.1, 11) -> (-18.1, 9) centre (-16.1, 9) ccw
  line L0 (-18.1, 9) -> (-18.1, -9)
  arc A1 (-18.1, -9) -> (-16.1, -11) centre (-16.1, -9) ccw
  line L1 (-16.1, -11) -> (18.1, -11)
  line L2 (18.1, -11) -> (18.1, 11)
  line L3 (18.1, 11) -> (-16.1, 11)
  circle A2 centre (4.79, 0) radius 1.91
  arc A3 (-9.66, -2.0302) -> (-6.1, -2.0302) centre (-7.88, 0) ccw
  line L4 (-9.66, -2.0302) -> (-9.66, 2.0302)
  arc A4 (-6.1, 2.0302) -> (-9.66, 2.0302) centre (-7.88, 0) ccw
  line L5 (-6.1, 2.0302) -> (-6.1, -2.0302)
  line L6 (-18.104, -8.5) -> (13.336, -8.5)
  circle A5 centre (13.336, -8.5) radius 1.5
  line L7 (13.336, -8.5) -> (13.336, 8.5)
  circle A6 centre (13.336, 8.5) radius 1.5
  dimension "d107" = 31.44
  dimension "d108" = 3
  dimension "d109" = 17
  dimension "d110" = 3
  constraint coincident L6.end A5.centre
  constraint perpendicular L6 L7
  constraint coincident L7.end A6.centre
  measures "d107" distance of L6.start L6.end
  measures "d108" diameter of A5
  measures "d109" distance of L6.end L7.end
  measures "d110" diameter of A6
extrude "Extrude21" cut sketch "Sketch27" against normal blind 20 contours L6 A5 L7 | L6 A5 L7 | A6 bodies 1

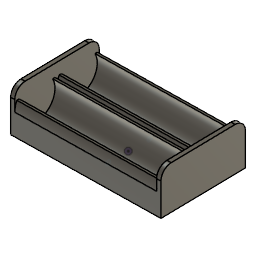
design "2x18650_holder"
part number: 2025-11-15-22-14-35-226
Autodesk Fusion 360 part; units mm, degrees
sketch "Sketch1" plane through (0, 0, 0) normal (0, 0, -1) x (1, 0, 0)
  circle A0 centre (0, 0) radius 9.225
  circle A1 centre (0, 0) radius 10.225
  line L0 (10.225, 10.225) -> (-10.225, 10.225)
  line L1 (-10.225, 10.225) -> (-10.225, 0)
  line L2 (10.225, 10.225) -> (10.225, 0)
  line L3 (10.225, 10.225) -> (7.503, 10.225)
  line L4 (7.503, 10.225) -> (7.503, -6.9466)
  line L5 (-7.5031, 10.225) -> (-10.225, 10.225)
  line L6 (-10.225, 10.225) -> (-7.5031, 10.225)
  line L7 (-7.5031, 10.225) -> (-7.5031, -6.9465)
  line L8 (-9.225, 10.225) -> (-9.225, 0)
  line L9 (9.225, 10.225) -> (9.225, 0)
  line L10 (10.225, 0) -> (9.225, 0)
  line L11 (9.225, 0) -> (9.225, 10.225)
  line L12 (9.0581, -4.7436) -> (0, 0)
  line L13 (0, 0) -> (-9.225, 4.4102)
  line L14 (9.0581, -4.7436) -> (-9.0581, -4.7436)
  line L15 (-9.0581, -4.7436) -> (0, 0)
  line L16 (0, 0) -> (8.8551, 5.1125)
  dimension "d1" = 20.45
  dimension "d2" = 2.722
  constraint coincident A0.centre A1.centre
  constraint horizontal L0
  constraint tangent A1 L0
  constraint perpendicular L0 L1
  constraint tangent A1 L1
  constraint perpendicular L0 L2
  constraint tangent A1 L2
  constraint coincident A1 L1.end
  constraint coincident L0 L5.start
  constraint perpendicular L2 L3
  constraint coincident A1 L4.end
  constraint perpendicular L3 L4
  constraint coincident A1 L7.end
  constraint perpendicular L0 L7
  constraint coincident L5 L8.start
  constraint perpendicular L6 L8
  constraint tangent A0 L8
  constraint coincident A0 L8.end
  constraint coincident L0 L9.start
  constraint perpendicular L0 L9
  constraint tangent A0 L9
  constraint coincident A0 L9.end
  constraint coincident A1 L12.start
  constraint coincident A1 L13.end
  constraint coincident L8 L13.end
  constraint coincident A1 L14.end
  constraint perpendicular L7 L14
  constraint coincident A1 L16.end
  measures "d1" diameter of A1
  measures "d2" distance of L0.start L3.end
sketch "Sketch2" plane through (0, 0, 0) normal (0, 0, -1) x (1, 0, 0)
  circle A0 centre (0, 0) radius 9.225
  circle A1 centre (0, 0) radius 10.225
  line L0 (0, -10.225) -> (-10.225, -10.225)
  line L1 (-10.225, -10.225) -> (-10.225, 10.225)
  line L2 (-10.225, 10.225) -> (0, 10.225)
  line L3 (4.4014, 9.2292) -> (4.4014, -9.2292)
  dimension "d5" = 20.45
  constraint concentric A0 A1
  constraint horizontal L0
  constraint vertical L1
  constraint horizontal L2
  constraint tangent A1 L1
  constraint tangent A1 L0
  constraint tangent A1 L2
  constraint coincident A1 L0.start
  constraint coincident A1 L2.end
  constraint coincident A1 L3.start
  constraint coincident A1 L3.end
  constraint vertical L3
  measures "d5" diameter of A1
extrude "Extrude2" add sketch "Sketch2" against normal blind 66.25 contours A0 A1 L3 | A1 L1 L2 | A1 L0 L1 picked at (0.6703, -9.8497)
mirror "Mirror1" about plane through (-5.1125, 10.225, 33.125) normal (0, 1, 0) of bodies 1 merged
sketch "Sketch3" plane through (0, 0, 66.25) normal (0, 0, 1) x (-1, 0, 0)
  arc A0 (-4.4014, -9.2292) -> (0, -10.225) centre (0, 0) ccw
  arc A1 (0, -10.225) -> (-4.4014, -11.2208) centre (0, -20.45) ccw
  line L0 (-4.4014, -11.2208) -> (-4.4014, -12.3427)
  arc A2 (-4.4014, -28.5573) -> (-4.4014, -12.3427) centre (0, -20.45) ccw
  line L1 (-4.4014, -28.5573) -> (-4.4014, -29.6792)
  arc A3 (-4.4014, -29.6792) -> (0, -30.675) centre (0, -20.45) ccw
  line L2 (0, -30.675) -> (10.225, -30.675)
  line L3 (10.225, -30.675) -> (10.225, 10.225)
  line L4 (10.225, 10.225) -> (0, 10.225)
  arc A4 (0, 10.225) -> (-4.4014, 9.2292) centre (0, 0) ccw
  line L5 (-4.4014, 9.2292) -> (-4.4014, 8.1073)
  arc A5 (-4.4014, -8.1073) -> (-4.4014, 8.1073) centre (0, 0) ccw
  line L6 (-4.4014, -8.1073) -> (-4.4014, -9.2292)
  line L7 (10.225, 10.225) -> (-5.225, 10.225)
  line L8 (-10.225, 5.225) -> (-10.225, -25.675)
  line L9 (-5.225, -30.675) -> (10.225, -30.675)
  line L10 (10.225, -30.675) -> (10.225, 10.225)
  arc A6 (-5.225, 10.225) -> (-10.225, 5.225) centre (-5.225, 5.225) ccw
  arc A7 (-10.225, -25.675) -> (-5.225, -30.675) centre (-5.225, -25.675) ccw
  point P0 (-10.225, 10.225)
  dimension "d11" = 20.45
  dimension "d12" = 40.9
  dimension "d13" = 5
  constraint horizontal L7
  constraint vertical L8
  constraint horizontal L9
  constraint vertical L10
  constraint coincident L3.end L4.start
  constraint coincident P0 L8
  constraint coincident P0 L7
  constraint tangent L8 A6
  constraint tangent L7 A6
  constraint tangent L8 A7
  constraint tangent L9 A7
  constraint equal A6 A7
  measures "d11" distance of L3.end P0
  measures "d12" distance of L3.end L2.end
  measures "d13" radius of A6
extrude "Extrude3" add sketch "Sketch3" along normal blind 2
sketch "Sketch4" plane through (0, 0, 0) normal (0, 0, -1) x (1, 0, 0)
  arc A0 (0, -10.225) -> (4.4014, -9.2292) centre (0, 0) ccw
  line L0 (4.4014, -9.2292) -> (4.4014, -8.1073)
  arc A1 (4.4014, 8.1073) -> (4.4014, -8.1073) centre (0, 0) ccw
  line L1 (4.4014, 8.1073) -> (4.4014, 9.2292)
  arc A2 (4.4014, 9.2292) -> (0, 10.225) centre (0, 0) ccw
  line L2 (0, 10.225) -> (-10.225, 10.225)
  line L3 (-10.225, 10.225) -> (-10.225, -30.675)
  line L4 (-10.225, -30.675) -> (0, -30.675)
  arc A3 (0, -30.675) -> (4.4014, -29.6792) centre (0, -20.45) ccw
  line L5 (4.4014, -29.6792) -> (4.4014, -28.5573)
  arc A4 (4.4014, -12.3427) -> (4.4014, -28.5573) centre (0, -20.45) ccw
  line L6 (4.4014, -12.3427) -> (4.4014, -11.2208)
  arc A5 (4.4014, -11.2208) -> (0, -10.225) centre (0, -20.45) ccw
  line L7 (-10.225, -30.675) -> (5.225, -30.675)
  line L8 (10.225, -25.675) -> (10.225, 5.225)
  line L9 (5.225, 10.225) -> (-10.225, 10.225)
  line L10 (-10.225, 10.225) -> (-10.225, -30.675)
  arc A6 (5.225, -30.675) -> (10.225, -25.675) centre (5.225, -25.675) ccw
  arc A7 (10.225, 5.225) -> (5.225, 10.225) centre (5.225, 5.225) ccw
  point P0 (10.225, -30.675)
  dimension "d16" = 20.45
  dimension "d17" = 40.9
  dimension "d18" = 5
  constraint horizontal L7
  constraint vertical L8
  constraint horizontal L9
  constraint vertical L10
  constraint coincident L3.end L4.start
  constraint coincident P0 L8
  constraint coincident P0 L7
  constraint tangent L8 A6
  constraint tangent L7 A6
  constraint tangent L8 A7
  constraint tangent L9 A7
  constraint equal A6 A7
  measures "d16" distance of L3.end P0
  measures "d17" distance of L3.end L2.end
  measures "d18" radius of A6
extrude "Extrude4" add sketch "Sketch4" along normal blind 2
move_body "Move1" bodies 1 to x (1, 0, 0) y (0, 1, 0) z (0, 0, 1) at (0, 0, 2)
sketch "Sketch5" plane through (-10.225, 0, 0) normal (-1, 0, 0) x (0, -1, 0)
  line L0 (10.225, 0) -> (10.225, 70.25)
  line L1 (10.225, 70.25) -> (-30.675, 70.25)
  line L2 (-30.675, 70.25) -> (-30.675, 0)
  line L3 (-30.675, 0) -> (10.225, 0)
  circle A0 centre (-20.45, 35.125) radius 1.25
  circle A1 centre (-0.7544, 35.125) radius 1.25
  line L4 (-20.45, 35.125) -> (-20.45, 62.125)
  line L5 (-20.45, 62.125) -> (-20.45, 8.125)
  line L6 (-0.7544, 35.125) -> (-0.7544, 62.125)
  line L7 (-0.7544, 62.125) -> (-0.7544, 8.125)
  circle A2 centre (-20.45, 8.125) radius 1.25
  circle A3 centre (-0.7544, 8.125) radius 1.25
  circle A4 centre (-20.45, 62.125) radius 1.25
  circle A5 centre (-0.7544, 62.125) radius 1.25
  point P0 (-20.45, 35.125)
  point P1 (-0.7544, 35.125)
  dimension "d26" = 2.5
  dimension "d27" = 2.5
  dimension "d28" = 27
  dimension "d29" = 54
  dimension "d30" = 27
  dimension "d31" = 54
  dimension "d32" = 2.5
  dimension "d33" = 2.5
  dimension "d34" = 2.5
  dimension "d35" = 2.5
  constraint coincident P0 A0.centre
  constraint coincident P1 A1.centre
  constraint parallel L2 L4
  constraint parallel L4 L5
  constraint vertical L6
  constraint parallel L6 L7
  constraint coincident L5.end A2.centre
  constraint coincident L7.end A3.centre
  constraint coincident L4.end L5.start
  constraint coincident L6.end L7.start
  measures "d26" diameter of A0
  measures "d27" diameter of A1
  measures "d28" distance of P0 L4.end
  measures "d29" distance of L4.end L5.end
  measures "d30" distance of P1 L6.end
  measures "d31" distance of L6.end L7.end
  measures "d32" diameter of A2
  measures "d33" diameter of A3
  measures "d34" diameter of A4
  measures "d35" diameter of A5
extrude "Extrude5" cut sketch "Sketch5" against normal blind 5 contours A0 L4 L5 | A0 L4 L5 | A1 L6 L7 | A1 L6 L7 | A2 | A3 | A4 | A5
sketch "Sketch6" plane through (-10.225, 0, 0) normal (-1, 0, 0) x (0, -1, 0)
sketch "Sketch7" plane through (-10.225, 0, 0) normal (-1, 0, 0) x (0, -1, 0)
sketch "Sketch8" plane through (-10.225, 0, 0) normal (-1, 0, 0) x (0, -1, 0)
move_body "Move2" bodies 1 to x (1, 0, 0) y (0, 1, 0) z (0, 0, 1) at (10.225, -10.3397, 0)
move_body "Move3" bodies 1 to x (1, 0, 0) y (0, 1, 0) z (0, 0, 1) at (0, 0, -35.125)
sketch "Sketch9" plane through (0, 0, 0) normal (-1, 0, 0) x (0, -1, 0)
  circle A0 centre (9.5853, 0) radius 1.25
  circle A1 centre (-10.1103, 0) radius 1.25
move_body "Move4" bodies 1 to x (0, 0, 1) y (-0.017452, 0.999848, 0) z (-0.999848, -0.017452, 0) at (-0.002, 0, 0)
